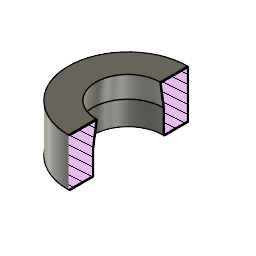
roket mount top 2 (Autodesk Fusion 360 design; units mm, degrees)
part number: 2026-05-01-17-27-18-302
Autodesk Fusion 360 part; units mm, degrees
sketch "Sketch4" plane through (0, 0, 0) normal (0, 0, 1) x (1, 0, 0)
  circle A0 centre (0, 0) radius 25 construction
  dimension "d8" = 50
  constraint coincident A0.centre origin
  measures "d8" diameter of A0
sketch "Sketch6" plane through (0, 0, 0) normal (1, 0, 0) x (0, 1, 0)
  line L0 (0, 0) -> (25, 0) construction
  line L1 (25, 0) -> (25, 10)
  line L2 (0, 0) -> (14.8, 0) construction
  line L3 (14.8, 0) -> (14.8, 10) construction
  line L4 (14.8, 10) -> (25, 10) construction
  line L5 (25, 10) -> (11.5, 10) construction
  line L6 (14.8, 0) -> (13.3946, 10) construction
  line L7 (14.8, 0) -> (24.8983, 0) construction
  line L8 (25, 10) -> (13.3946, 10)
  line L9 (13.3946, 10) -> (14.8, 0)
  line L10 (25, 0) -> (14.8, 0)
  dimension "d9" = 25
  dimension "d10" = 10
  dimension "d11" = 14.8
  dimension "d12" = 98
  constraint coincident L0.start L2.start
  constraint horizontal L0
  constraint perpendicular L0 L1
  constraint parallel L0 L2
  constraint perpendicular L2 L3
  constraint perpendicular L3 L5
  constraint horizontal L7
  constraint coincident L5 L6.end
  measures "d9" distance of L0.start L0.end
  measures "d10" distance of L0.end L1.end
  measures "d11" distance of L0.start L2.end
  measures "d12" angle of L6 L7
revolve "Revolve1" add sketch "Sketch6" angle 360 about axis through (0, 0, 1.75) along (0, 0, 1)
sketch "Sketch7" plane through (0, 0, 0) normal (0, 0, -1) x (1, 0, 0)
  circle A0 centre (0, 0) radius 25
  circle A1 centre (0, 0) radius 14.8
extrude "Extrude3" add 1 faces at (1.9773, 21.4518, 0) along direction (0, 0, -1) blind 10
